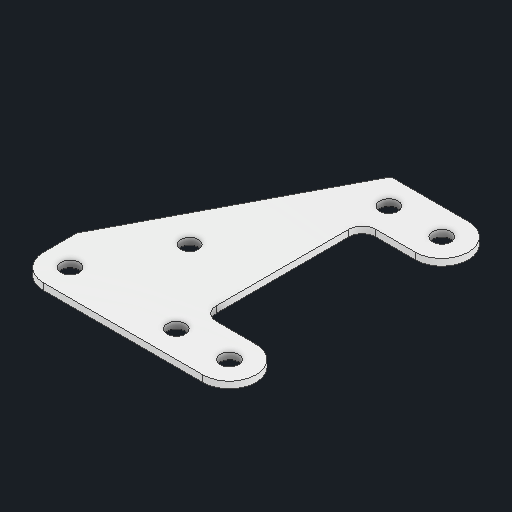
# Autodesk Inventor part: gusset
Saved by Autodesk Inventor 2025 (Build 290162000, 162)
## iProperties
Created: 2024-06-18
Part Number: gusset
Material: Acetal Resin, White
Document SubType Name: Modeling
Designer: Averey Ku
Density: 1.425 g/cm^3
Appearance: Smooth - White
d0: 0.125 in
d3: 0.165 in
Author: Averey Ku
Autodesk Inventor part; units mm, degrees
ref_plane "YZ Plane" through (0, 0, 0) normal (1, 0, 0) x (0, 1, 0)
ref_plane "XZ Plane" through (0, 0, 0) normal (0, 1, 0) x (-1, 0, 0)
ref_plane "XY Plane" through (0, 0, 0) normal (0, 0, 1) x (1, 0, 0)
sketch "main" plane through (0, 0, 0) normal (0, 0, 1) x (1, 0, 0)
  circle A0 centre (18.656, 25.5497) radius 2.1844
  circle A1 centre (-6.744, 25.5497) radius 2.1844
  line L0 (-6.744, 16.0247) -> (-6.744, -15.7253)
  line L1 (-0.394, -30.5843) -> (25.006, 17.6122)
  arc A2 (-6.744, 16.0247) -> (-9.919, 19.1997) centre (-9.919, 16.0247) ccw
  line L2 (-19.444, 19.1997) -> (-9.919, 19.1997)
  circle A3 centre (-19.444, 25.5497) radius 2.1844
  arc A4 (-19.444, 31.8997) -> (-19.444, 19.1997) centre (-19.444, 25.5497) ccw
  line L3 (25.006, 25.5497) -> (25.006, 17.6122)
  line L4 (18.656, 31.8997) -> (-19.444, 31.8997)
  arc A5 (25.006, 25.5497) -> (18.656, 31.8997) centre (18.656, 25.5497) ccw
  arc A6 (-9.919, -18.9003) -> (-6.744, -15.7253) centre (-9.919, -15.7253) ccw
  line L5 (-19.444, -18.9003) -> (-9.919, -18.9003)
  circle A7 centre (-6.744, -25.2503) radius 2.1844
  line L6 (-0.394, -30.5843) -> (-1.41, -31.6003)
  circle A8 centre (-19.444, -25.2503) radius 2.1844
  arc A9 (-19.444, -18.9003) -> (-19.444, -31.6003) centre (-19.444, -25.2503) ccw
  line L7 (-1.41, -31.6003) -> (-19.444, -31.6003)
  circle A10 centre (9.131, 6.4997) radius 2.0955
  point P0 (-4.4485, 2.2347)
  dimension "d0" = 3.175
  dimension "d3" = 4.191
  measures "d0" radius of A2
  measures "d3" diameter of A10
sketch "Sketch1" plane through (0, 0, 0) normal (0, 1, 0) x (-1, 0, 0)
  circle A0 centre (38.1, 0) radius 2.1844
  circle A1 centre (12.7, 0) radius 2.1844
  line L0 (12.7, -9.525) -> (12.7, -41.275)
  line L1 (19.05, -56.134) -> (44.45, -7.9375)
  arc A2 (12.7, -9.525) -> (9.525, -6.35) centre (9.525, -9.525) ccw
  line L2 (0, -6.35) -> (9.525, -6.35)
  circle A3 centre (0, 0) radius 2.1844
  arc A4 (0, 6.35) -> (0, -6.35) centre (0, 0) ccw
  line L3 (44.45, 0) -> (44.45, -7.9375)
  line L4 (38.1, 6.35) -> (0, 6.35)
  arc A5 (44.45, 0) -> (38.1, 6.35) centre (38.1, 0) ccw
  arc A6 (9.525, -44.45) -> (12.7, -41.275) centre (9.525, -41.275) ccw
  line L5 (0, -44.45) -> (9.525, -44.45)
  circle A7 centre (12.7, -50.8) radius 2.1844
  line L6 (19.05, -56.134) -> (18.034, -57.15)
  circle A8 centre (0, -50.8) radius 2.1844
  arc A9 (0, -44.45) -> (0, -57.15) centre (0, -50.8) ccw
  line L7 (18.034, -57.15) -> (0, -57.15)
  circle A10 centre (28.575, -19.05) radius 2.0955
  constraints: 1 other
extrude "Extrusion1" add sketch "Sketch1" along normal blind 1.5875
body "Solid1"
